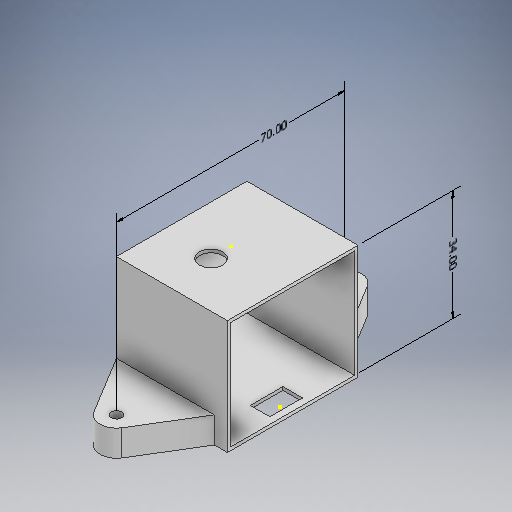
# Autodesk Inventor part: SERVO BASE HOUSING
Saved by Autodesk Inventor 2025.3 (Build 293356000, 356)
## iProperties
Created: 2026-04-19
Part Number: SERVO BASE HOUSING
Material: Generic
Document SubType Name: Modeling
Designer: youse
Density: 1 g/cm^3
Appearance: Default
Author: youse
## iProperties of the stored document SERVO BASE HOUSING_3DPrint.ipt
Created: 2026-05-01
Part Number: SERVO BASE HOUSING_3DPrint
Material: Generic
Document SubType Name: Modeling
Designer: youse
Density: 1 g/cm^3
Appearance: Default
Author: youse
Autodesk Inventor part; units mm, degrees
ref_plane "YZ Plane" through (0, 0, 0) normal (1, 0, 0) x (0, 1, 0)
ref_plane "XZ Plane" through (0, 0, 0) normal (0, 1, 0) x (-1, 0, 0)
ref_plane "XY Plane" through (0, 0, 0) normal (0, 0, 1) x (1, 0, 0)
sketch "Sketch1" plane through (0, 0, 0) normal (0, 1, 0) x (-1, 0, 0)
  line L0 (-15, 20) -> (15, 20)
  line L1 (15, 20) -> (15, -20)
  line L2 (15, -20) -> (-15, -20)
  line L3 (-15, -20) -> (-15, 20)
  line L4 (-15, 20) -> (15, -20) construction
  line L5 (15, 20) -> (-15, -20) construction
  line L6 (0, 31.25) -> (0, -31.25)
  point P0 (0, 0)
  dimension "d0" = 30
  dimension "d1" = 40
  dimension "d2" = 62.5
  dimension "d3" = 18.75
  constraints: 14 end point, 3 midpoint, 2 parallel, 1 horizontal, 1 perpendicular, 1 vertical
  measures "d0" distance of L1.end L2.end
  measures "d1" distance of L2.end L0.start
  measures "d2" distance of L6.start L6.end
  measures "d3" distance from line of L6.start L5
extrude "Extrusion1" add sketch "Sketch1" along normal blind 35
shell "Shell1" thickness 1 removed faces 1 at (15, 11.6667, 6.6667)
sketch "Sketch3" plane through (0, 35, 0) normal (0, 1, 0) x (1, 0, 0)
  point P0 (0, 0)
sketch "Sketch4" plane through (0, 0, 0) normal (0, 1, 0) x (-1, 0, 0)
  arc A0 (-4.2693, -37.6026) -> (4.2693, -37.6026) centre (0, -35) ccw
  line L0 (-15, -20) -> (15, -20) projected
  line L1 (28.6058, 0) -> (-27.8274, 0)
  line L2 (15, -20) -> (15, 20) projected
  arc A1 (4.2693, 37.6026) -> (-4.2693, 37.6026) centre (0, 35) ccw
  line L3 (15, -20) -> (4.2693, -37.6026)
  line L4 (-15, -20) -> (-4.2693, -37.6026)
  line L5 (15, 20) -> (-15, 20) projected
  line L6 (-15, 20) -> (-4.2693, 37.6026)
  line L7 (15, 20) -> (4.2693, 37.6026)
  circle A2 centre (0, -35) radius 1.6
  circle A3 centre (0, 35) radius 1.6
  point P0 (0, 0)
  point P1 (0, -20)
  point P2 (0.3892, 0)
  point P3 (15, 0)
  dimension "d7" = 10
  dimension "d8" = 15
  dimension "d9" = 3.2
  dimension "d10" = 3.2
  constraints: 10 end point, 4 centre point, 4 point on circle, 4 tangent, 3 midpoint, 2 coincident, 1 horizontal, 1 horizontal alignment, 1 symmetric about line, 1 vertical alignment, 1 other
  measures "d7" diameter of A0
  measures "d8" distance of point (0, -20) A0.centre
  measures "d9" diameter of A2
  measures "d10" diameter of A3
extrude "Extrusion2" add sketch "Sketch4" along normal blind 8
sketch "Sketch5" plane through (0, 35, 0) normal (0, 1, 0) x (1, 0, 0)
  circle A0 centre (0, -6) radius 3.55
  point P0 (0, 0)
  dimension "d15" = 7.1
  dimension "d16" = 6
  constraints: 1 centre point, 1 vertical alignment
  measures "d15" diameter of A0
  measures "d16" distance of A0.centre point (0, 0)
extrude "Extrusion3" cut sketch "Sketch5" against normal blind 10
sketch "Sketch6" plane through (15, 0, 20) normal (1, 0, 0) x (0, 0, -1)
  point P0 (20, 0)
sketch "Sketch7" plane through (15, 35, 20) normal (1, 0, 0) x (0, 0, -1)
  line L0 (0, -27) -> (0, 0) projected
  line L1 (40, -35) -> (0, -35)
  line L2 (0, -35) -> (0, 0)
  line L3 (0, 0) -> (40, 0)
  line L4 (40, 0) -> (40, -35)
  line L5 (40, -35) -> (0, 0) construction
  line L6 (0, -35) -> (40, 0) construction
  line L7 (1, -34) -> (1, -1) projected
  line L8 (0, 0) -> (40, 0) projected
  line L9 (1, -1) -> (39, -1) projected
  line L10 (1, -34) -> (39, -34)
  line L11 (39, -34) -> (39, -1)
  line L12 (39, -1) -> (1, -1)
  line L13 (1, -1) -> (1, -34)
  line L14 (1, -34) -> (39, -1) construction
  line L15 (39, -34) -> (1, -1) construction
  point P0 (20, -35)
  point P1 (0, -25)
  point P2 (20, -17.5)
  point P3 (20, 0)
  point P4 (1, -17.5)
  point P5 (0, -17.5)
  point P6 (20, -35)
  point P7 (20, 0)
  point P8 (0, -25)
  constraints: 24 end point, 9 midpoint, 4 parallel, 2 horizontal, 2 perpendicular, 2 vertical alignment, 1 horizontal alignment
extrude "Extrusion4" add sketch "Sketch7" along normal blind 4
sketch "Sketch9" plane through (-14, 1, 19) normal (0, 1, 0) x (1, 0, 0)
  line L0 (25, 24) -> (31, 24)
  line L1 (31, 24) -> (31, 14)
  line L2 (31, 14) -> (25, 14)
  line L3 (25, 14) -> (25, 24)
  line L4 (25, 24) -> (31, 14) construction
  line L5 (31, 24) -> (25, 14) construction
  line L6 (33, 38) -> (33, 0) projected
  point P0 (14, 19)
  point P1 (28, 19)
  point P2 (33, 19)
  point P3 (33, 19)
  dimension "d25" = 6
  dimension "d26" = 10
  dimension "d27" = 5
  constraints: 12 end point, 4 midpoint, 2 parallel, 1 horizontal, 1 horizontal alignment, 1 perpendicular
  measures "d25" distance of L1.end L2.end
  measures "d26" distance of L0.end L1.end
  measures "d27" distance of point (33, 19) point (28, 19)
extrude "Extrusion6" cut sketch "Sketch9" against normal through all
body "Solid1"
